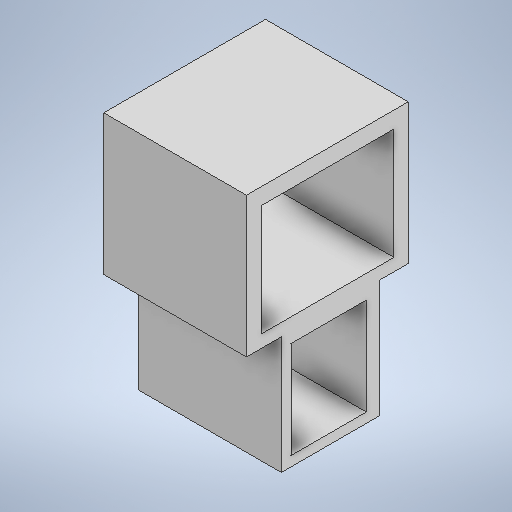
# Autodesk Inventor part: Part1
Saved by Autodesk Inventor 2025.1 (Build 291241000, 241)
## iProperties
Created: 2025-09-12
Part Number: Part1
Material: Generic
Document SubType Name: Modeling
Designer: nbro174
Density: 1 g/cm^3
Appearance: Default
Author: nbro174
Autodesk Inventor part; units mm, degrees
ref_plane "YZ Plane" through (0, 0, 0) normal (1, 0, 0) x (0, 1, 0)
ref_plane "XZ Plane" through (0, 0, 0) normal (0, 1, 0) x (-1, 0, 0)
ref_plane "XY Plane" through (0, 0, 0) normal (0, 0, 1) x (1, 0, 0)
sketch "Sketch1" plane through (0, 0, 0) normal (1, 0, 0) x (0, 1, 0)
  line L0 (13.6162, 14.8297) -> (-11.3125, 14.8297)
  line L1 (-11.3125, 14.8297) -> (-11.3125, -13.9659)
  line L2 (-11.3125, -13.9659) -> (13.6162, -13.9659)
  line L3 (13.6162, -13.9659) -> (13.6162, 14.8297)
  constraints: 8 end point, 2 parallel, 1 horizontal, 1 perpendicular
extrude "Extrusion1" add sketch "Sketch1" along normal mid plane 25.4
sketch "Sketch2" plane through (12.7, 0, 0) normal (1, 0, 0) x (0, 0, -1)
  line L0 (-12.1558, 10.6955) -> (11.4154, 10.6955)
  line L1 (11.4154, 10.6955) -> (11.4154, -9.0912)
  line L2 (11.4154, -9.0912) -> (-12.1558, -9.0912)
  line L3 (-12.1558, -9.0912) -> (-12.1558, 10.6955)
  point P0 (0, 0)
  constraints: 8 end point, 2 parallel, 1 horizontal, 1 perpendicular
extrude "Extrusion2" cut sketch "Sketch2" against normal blind 25.4
sketch "Sketch3" plane through (12.7, 0, 0) normal (1, 0, 0) x (0, 0, -1)
  line L0 (-14.8297, -11.3125) -> (13.9659, -11.3125) projected
  line L1 (-8.621, -11.3125) -> (8.8651, -11.3125)
  line L2 (8.8651, -11.3125) -> (8.8651, -32.2195)
  line L3 (8.8651, -32.2195) -> (-8.621, -32.2195)
  line L4 (-8.621, -32.2195) -> (-8.621, -11.3125)
  point P0 (0, 0)
  constraints: 8 end point, 2 parallel, 1 horizontal, 1 perpendicular, 1 point on line
extrude "Extrusion3" add sketch "Sketch3" against normal blind 25.4
sketch "Sketch4" plane through (12.7, 0, 0) normal (1, 0, 0) x (0, 0, -1)
  line L0 (-6.8955, -13.2073) -> (6.5094, -13.2073)
  line L1 (6.5094, -13.2073) -> (6.5094, -30.471)
  line L2 (6.5094, -30.471) -> (-6.8955, -30.471)
  line L3 (-6.8955, -30.471) -> (-6.8955, -13.2073)
  point P0 (0, 0)
  constraints: 8 end point, 2 parallel, 1 horizontal, 1 perpendicular
extrude "Extrusion4" cut sketch "Sketch4" against normal blind 25.4
sketch "Sketch6" plane through (12.7, -32.2195, -8.8651) normal (0, -1, 0) x (1, 0, 0)
  point P0 (-12.7, 8.8651)
body "Solid1"
